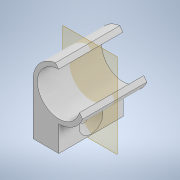
# Autodesk Inventor part: shadeHolderV02
Saved by Autodesk Inventor 2021.2 (Build 252289000, 289)
## iProperties
Created: 2021-02-12
Part Number: shadeHolderV02
Material: Generic
Document SubType Name: Modeling
Designer: robst
Density: 1 g/cm^3
Appearance: Default
Author: robst
Autodesk Inventor part; units mm, degrees
ref_plane "YZ Plane" through (0, 0, 0) normal (1, 0, 0) x (0, 1, 0)
ref_plane "XZ Plane" through (0, 0, 0) normal (0, 1, 0) x (-1, 0, 0)
sketch "Sketch4" plane through (0, 0, 0) normal (0, 0, 1) x (1, 0, 0)
  arc A0 (-0.0698, 6.3496) -> (6.1152, -1.7109) centre (0, 0) ccw
  arc A1 (-0.9946, 7.5548) -> (7.04, -2.916) centre (0, 0) ccw
  line L0 (0, 0) -> (0, 7.9375) construction
  line L1 (-0.0698, 6.3496) -> (6.1152, -1.7109) construction
  line L2 (-0.0698, 6.3496) -> (-0.9946, 7.5548)
  line L3 (6.1152, -1.7109) -> (7.04, -2.916)
  circle A2 centre (0, 0) radius 6.35
  dimension "d10" = 12.7
  dimension "d11" = 1.27
  dimension "d12" = 37.5
  dimension "d13" = 10.16
  constraints: 8 end point, 4 point on circle, 3 centre point, 3 coincident, 1 collinear, 1 concentric, 1 point on line, 1 vertical
  measures "d10" diameter of A0
  measures "d11" radial gap between concentric circles of A1 A0
  measures "d12" angle of L1 L0
  measures "d13" distance of L1.start L1.end
extrude "Extrusion3" add sketch "Sketch4" along normal mid plane 19.05 contours A0 L3 A1 L2
sketch "Sketch5" plane through (0, 0, 0) normal (0, 0, 1) x (1, 0, 0)
  arc A0 (-0.9946, 7.5548) -> (7.04, -2.916) centre (0, 0) ccw projected
  line L0 (-7.62, 0) -> (-7.62, -15.24)
  line L1 (-7.62, -15.24) -> (0, -15.24)
  line L2 (0, -15.24) -> (0, -7.62)
  circle A1 centre (0, 0) radius 7.9375
  dimension "d16" = 7.62
  constraints: 6 end point, 2 perpendicular, 2 point on circle, 1 centre point, 1 coincident, 1 tangent, 1 vertical
  measures "d16" distance from line of L2.end L1
extrude "Extrusion4" add sketch "Sketch5" along normal mid plane 19.05 contours A0 L2 A1 L0 | A1 L2 L1 L0 picked at (-7.3048, -2.4081)
sketch "Sketch6" plane through (0, -15.24, 9.525) normal (1, 0, 0) x (0, 0, -1)
  line L0 (0, 7.62) -> (19.05, 7.62) projected
  line L1 (19.05, 7.62) -> (19.05, 0) projected
  line L2 (0, 0) -> (19.05, 0) projected
  line L3 (0, 0) -> (0, 7.62) projected
  line L4 (0, 7.62) -> (19.05, 0) construction
  line L5 (19.05, 7.62) -> (0, 0) construction
  point P0 (9.525, 15.24)
  point P1 (9.525, 3.81)
  constraints: 4 end point, 1 midpoint
hole "Hole1" at (0, -11.43, 0) direction (-1, 0, 0) diameter 3.5052 end through all countersink diameter 7.112 countersink angle 82
sketch "Sketch10" plane through (-7.62, -15.24, 9.525) normal (0, -1, 0) x (1, 0, 0)
  line L0 (0, -19.05) -> (0, 0) projected
  line L1 (7.62, -19.05) -> (0, -19.05) projected
  line L2 (7.62, 0) -> (7.62, -19.05) projected
  line L3 (0, 0) -> (7.62, 0) projected
  line L4 (3.81, -19.05) -> (3.81, 0) construction
  spline S0 degree 2 poles (2.8014, -11.7171) (3.1307, -11.7171) (3.7235, -11.9518) (3.9294, -12.1617) knots 0 0 0 1 2 2 2
  spline S1 degree 2 poles (3.9294, -12.1617) (4.1887, -12.4252) (4.4563, -13.1374) (4.4563, -13.6808) knots 0 0 0 1 2 2 2
  line L5 (4.4563, -13.6808) -> (4.4563, -14.253)
  line L6 (4.4563, -14.253) -> (6.35, -14.253)
  line L7 (6.35, -14.253) -> (6.35, -14.9282)
  line L8 (6.35, -14.9282) -> (1.27, -14.9282)
  line L9 (1.27, -14.9282) -> (1.27, -13.652)
  spline S2 degree 2 poles (1.27, -13.652) (1.27, -13.1991) (1.4182, -12.5652) (1.587, -12.3223) knots 0 0 0 1 2 2 2
  spline S3 degree 2 poles (1.587, -12.3223) (1.7805, -12.0382) (2.3774, -11.7171) (2.8014, -11.7171) knots 0 0 0 1 2 2 2
  spline S4 degree 2 poles (2.822, -12.4211) (2.5585, -12.4211) (2.1716, -12.6022) (2.0481, -12.7875) knots 0 0 0 1 2 2 2
  spline S5 degree 2 poles (2.0481, -12.7875) (1.941, -12.948) (1.8546, -13.3762) (1.8546, -13.6932) knots 0 0 0 1 2 2 2
  line L10 (1.8546, -13.6932) -> (1.8546, -14.253)
  line L11 (1.8546, -14.253) -> (3.88, -14.253)
  line L12 (3.88, -14.253) -> (3.88, -13.792)
  spline S6 degree 2 poles (3.88, -13.792) (3.88, -13.3803) (3.7482, -12.8739) (3.5753, -12.7093) knots 0 0 0 1 2 2 2
  spline S7 degree 2 poles (3.5753, -12.7093) (3.423, -12.5569) (3.0649, -12.4211) (2.822, -12.4211) knots 0 0 0 1 2 2 2
  line L13 (1.27, -7.3905) -> (6.35, -9.1401)
  line L14 (6.35, -9.1401) -> (6.35, -9.8687)
  line L15 (6.35, -9.8687) -> (1.27, -11.6183)
  line L16 (1.27, -11.6183) -> (1.27, -10.8938)
  line L17 (1.27, -10.8938) -> (5.4896, -9.4859)
  line L18 (5.4896, -9.4859) -> (1.27, -8.078)
  line L19 (1.27, -8.078) -> (1.27, -7.3905)
  line L20 (4.6045, -3.7225) -> (4.6045, -4.3277)
  line L21 (4.6045, -4.3277) -> (6.35, -4.3277)
  line L22 (6.35, -4.3277) -> (6.35, -4.9822)
  line L23 (6.35, -4.9822) -> (4.6045, -4.9822)
  line L24 (4.6045, -4.9822) -> (4.6045, -7.2258)
  line L25 (4.6045, -7.2258) -> (3.8882, -7.2258)
  line L26 (3.8882, -7.2258) -> (1.27, -4.9534)
  line L27 (1.27, -4.9534) -> (1.27, -4.3277)
  line L28 (1.27, -4.3277) -> (4.057, -4.3277)
  line L29 (4.057, -4.3277) -> (4.057, -3.7225)
  line L30 (4.057, -3.7225) -> (4.6045, -3.7225)
  line L31 (4.057, -4.9822) -> (2.0728, -4.9822)
  line L32 (2.0728, -4.9822) -> (4.057, -6.6907)
  line L33 (4.057, -6.6907) -> (4.057, -4.9822)
  point P0 (7.62, -9.525)
  constraints: 2 end point, 2 midpoint, 1 vertical
extrude "Text" cut sketch "Sketch10" against normal blind 1.143 contours S0 S1 L5 L6 L7 L8 L9 S2 S3 | L13 L14 L15 L16 L17 L18 L19 | L20 L21 L22 L23 L24 L25 L26 L27 L28 L29 L30
equation "\"d10\" = shadeDiameter"
equation "\"d11\" = shadeHolderWallThickness"
equation "\"d13\" = openingForShade"
equation "\"d14\" = partWidth"
equation "\"d16\" = flatBelowShade"
equation "\"d17\" = partWidth"
equation "\"d28\" = textDepth"
equation "\"shadeDiameter\" = 12.7"
equation "\"partWidth\" = 19.05"
equation "\"backThickness\" = 1.905"
equation "\"backHeight\" = 25.4"
equation "\"cutTiltAngle\" = 52.5deg"
equation "\"flatBelowShade\" = 7.62"
equation "\"shadeHolderWallThickness\" = 1.27"
equation "\"openingForShade\" = 10.16"
equation "\"textDepth\" = 1.143"
body "Solid2"
